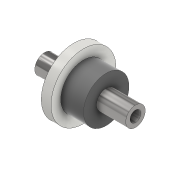
# Autodesk Inventor part: dfifferential
Saved by Autodesk Inventor 2022 (Build 260153000, 153)
## iProperties
Created: 2024-03-23
Part Number: dfifferential
Material: Generic
Document SubType Name: Modeling
Designer: david
Density: 1 g/cm^3
Appearance: Default
Author: david
Autodesk Inventor part; units mm, degrees
ref_plane "XZ Plane" through (0, 0, 0) normal (0, 1, 0) x (-1, 0, 0)
ref_plane "XY Plane" through (0, 0, 0) normal (0, 0, 1) x (1, 0, 0)
sketch "Sketch1" plane through (0, 0, 0) normal (1, 0, 0) x (0, 1, 0)
  circle A0 centre (0, 0) radius 4.5
  dimension "d0" = 9
  constraints: 1 centre point, 1 coincident
  measures "d0" diameter of A0
extrude "Extrusion1" add sketch "Sketch1" along normal mid plane 42
sketch "Sketch2" plane through (21, 0, 0) normal (1, 0, 0) x (0, 0, -1)
  circle A0 centre (0, 0) radius 4.5 projected
  constraints: 1 coincident
hole "Hole1" at (21, 0, 0) direction (-1, 0, 0) diameter 5 depth 7 tip angle 118
mirror "Mirror1" about plane through (0, 0, 0) normal (1, 0, 0) of "Hole1"
ref_plane "Work Plane2" through (-7.5, 0, 0) normal (1, 0, 0) x (0, 1, 0)
sketch "Sketch3" plane through (-7.5, 0, 0) normal (1, 0, 0) x (0, 1, 0)
  circle A0 centre (0, 0) radius 15
  dimension "d10" = 30
  constraints: 1 centre point, 1 coincident
  measures "d10" diameter of A0
extrude "Extrusion2" add sketch "Sketch3" along normal blind 4.5
sketch "Sketch4" plane through (-7.5, 0, 0) normal (-1, 0, 0) x (0, 0, 1)
  circle A0 centre (0, 0) radius 10.5
  dimension "d13" = 21
  constraints: 1 centre point, 1 coincident
  measures "d13" diameter of A0
extrude "Extrusion3" add sketch "Sketch4" against normal blind 15
body "Solid1"
